Autodesk Fusion 360 part; units mm, degrees
(part 4 of 8)
  spline S98 degree 5 poles (306.7756, -389.774) (306.6868, -389.747) (306.5093, -389.6931) (306.243, -389.6127) (305.8878, -389.5066) (305.4436, -389.3756) (304.9994, -389.2464) (304.5549, -389.1189) (304.1104, -388.9931) (303.6657, -388.869) (303.2209, -388.7467) (302.776, -388.6262) (302.3309, -388.5074) (301.8858, -388.3905) (301.4405, -388.2753) (300.9951, -388.162) (300.5496, -388.0505) (300.1041, -387.9408) (299.6584, -387.833) (299.2127, -387.7271) (298.7668, -387.623) (298.3209, -387.5209) (297.875, -387.4207) (297.4289, -387.3224) (296.9828, -387.2261) (296.5366, -387.1317) (296.0904, -387.0393) (295.6441, -386.949) (295.1978, -386.8606) (294.7515, -386.7743) (294.3051, -386.6901) (293.8587, -386.6079) (293.4123, -386.5279) (292.9659, -386.45) (292.5194, -386.3742) (292.073, -386.3006) (291.6266, -386.2292) (291.1802, -386.1601) (290.7338, -386.0932) (290.2874, -386.0286) (289.8411, -385.9663) (289.3949, -385.9064) (288.9486, -385.8488) (288.5025, -385.7937) (288.0564, -385.741) (287.6104, -385.6908) (287.1645, -385.6431) (286.7186, -385.5981) (286.273, -385.5557) (285.8274, -385.5159) (285.3819, -385.4789) (284.9366, -385.4446) (284.4915, -385.4131) (284.0465, -385.3845) (283.6017, -385.3588) (283.1571, -385.3362) (282.7128, -385.3169) (282.2687, -385.3009) (281.825, -385.2883) (281.3815, -385.2792) (280.9383, -385.2735) (280.4954, -385.2712) (280.0528, -385.2725) (279.6543, -385.277) (279.3446, -385.2831) (279.1234, -385.2889) (278.9906, -385.2929) (278.9461, -385.2943) knots -1 -1 -1 -1 -1 -1 -0.98571429 -0.97142857 -0.95714286 -0.94285714 -0.92857143 -0.91428571 -0.9 -0.88571429 -0.87142857 -0.85714286 -0.84285714 -0.82857143 -0.81428571 -0.8 -0.78571429 -0.77142857 -0.75714286 -0.74285714 -0.72857143 -0.71428571 -0.7 -0.68571429 -0.67142857 -0.65714286 -0.64285714 -0.62857143 -0.61428571 -0.6 -0.58571429 -0.57142857 -0.55714286 -0.54285714 -0.52857143 -0.51428571 -0.5 -0.48571429 -0.47142857 -0.45714286 -0.44285714 -0.42857143 -0.41428571 -0.4 -0.38571429 -0.37142857 -0.35714286 -0.34285714 -0.32857143 -0.31428571 -0.3 -0.28571429 -0.27142857 -0.25714286 -0.24285714 -0.22857143 -0.21428571 -0.2 -0.18571429 -0.17142857 -0.15714286 -0.14285714 -0.12857143 -0.11428571 -0.10707295 -0.10707295 -0.10707295 -0.10707295 -0.10707295 -0.10707295
  spline S99 degree 3 poles (277.3377, -384.0136) (277.3775, -384.2165) (277.4566, -384.4096) (277.6843, -384.7546) (277.8308, -384.9033) (278.1397, -385.1137) (278.2917, -385.1853) (278.6124, -385.2786) (278.7791, -385.2997) (278.9461, -385.2943) knots 0 0 0 0 0.062015 0.062015 0.12403 0.12403 0.174133 0.174133 0.224236 0.224236 0.224236 0.224236
  arc A50 (277.3377, -384.0136) -> (275.5948, -375.8142) centre (11.949, -436.1388) ccw
  spline S100 degree 3 poles (276.5432, -373.99) (276.3518, -374.068) (276.1774, -374.1826) (275.8825, -374.4723) (275.7647, -374.6446) (275.6175, -374.9881) (275.5763, -375.151) (275.5463, -375.4837) (275.5576, -375.6514) (275.5948, -375.8142) knots 0 0 0 0 0.062015 0.062015 0.12403 0.12403 0.174133 0.174133 0.224236 0.224236 0.224236 0.224236
  spline S101 degree 5 poles (276.5432, -373.99) (276.5845, -373.9731) (276.7075, -373.9228) (276.9119, -373.8381) (277.1973, -373.7177) (277.5632, -373.5598) (277.968, -373.3809) (278.3717, -373.1987) (278.7743, -373.0133) (279.1757, -372.8245) (279.576, -372.6325) (279.9752, -372.4373) (280.3732, -372.2389) (280.7702, -372.0374) (281.1661, -371.8331) (281.5609, -371.6259) (281.9548, -371.4161) (282.3476, -371.2036) (282.7395, -370.9886) (283.1304, -370.7711) (283.5203, -370.5511) (283.9093, -370.3286) (284.2972, -370.1037) (284.6843, -369.8764) (285.0703, -369.6468) (285.4555, -369.415) (285.8397, -369.1809) (286.223, -368.9446) (286.6054, -368.7062) (286.9869, -368.4656) (287.3675, -368.223) (287.7472, -367.9783) (288.126, -367.7315) (288.5039, -367.4827) (288.8809, -367.2319) (289.2571, -366.9791) (289.6324, -366.7244) (290.0067, -366.4678) (290.3803, -366.2093) (290.7529, -365.9489) (291.1247, -365.6867) (291.4956, -365.4226) (291.8657, -365.1567) (292.2349, -364.889) (292.6033, -364.6196) (292.9708, -364.3484) (293.3374, -364.0754) (293.7033, -363.8008) (294.0682, -363.5244) (294.4324, -363.2463) (294.7956, -362.9666) (295.1581, -362.6851) (295.5197, -362.4021) (295.8805, -362.1174) (296.2404, -361.8311) (296.5995, -361.5432) (296.9578, -361.2537) (297.3152, -360.9626) (297.6718, -360.67) (298.0276, -360.3758) (298.3825, -360.08) (298.7367, -359.7828) (299.09, -359.484) (299.4424, -359.1837) (299.7238, -358.9423) (299.9344, -358.7605) (300.0746, -358.6391) (300.1447, -358.5783) knots 0.10707295 0.10707295 0.10707295 0.10707295 0.10707295 0.10707295 0.11428571 0.12857143 0.14285714 0.15714286 0.17142857 0.18571429 0.2 0.21428571 0.22857143 0.24285714 0.25714286 0.27142857 0.28571429 0.3 0.31428571 0.32857143 0.34285714 0.35714286 0.37142857 0.38571429 0.4 0.41428571 0.42857143 0.44285714 0.45714286 0.47142857 0.48571429 0.5 0.51428571 0.52857143 0.54285714 0.55714286 0.57142857 0.58571429 0.6 0.61428571 0.62857143 0.64285714 0.65714286 0.67142857 0.68571429 0.7 0.71428571 0.72857143 0.74285714 0.75714286 0.77142857 0.78571429 0.8 0.81428571 0.82857143 0.84285714 0.85714286 0.87142857 0.88571429 0.9 0.91428571 0.92857143 0.94285714 0.95714286 0.97142857 0.98571429 1 1 1 1 1 1
  arc A51 (300.1447, -358.5783) -> (297.4536, -349.1933) centre (11.949, -436.1388) ccw
  spline S102 degree 5 poles (297.4536, -349.1933) (297.362, -349.1789) (297.1787, -349.1502) (296.9037, -349.1077) (296.5372, -349.052) (296.0792, -348.9842) (295.6212, -348.918) (295.1634, -348.8536) (294.7057, -348.7909) (294.2481, -348.7299) (293.7906, -348.6707) (293.3332, -348.6133) (292.8759, -348.5576) (292.4188, -348.5037) (291.9619, -348.4517) (291.5051, -348.4014) (291.0484, -348.353) (290.5919, -348.3064) (290.1356, -348.2617) (289.6794, -348.2188) (289.2235, -348.1779) (288.7677, -348.1388) (288.3121, -348.1016) (287.8567, -348.0664) (287.4015, -348.033) (286.9466, -348.0017) (286.4918, -347.9723) (286.0373, -347.9449) (285.5831, -347.9196) (285.1291, -347.8962) (284.6753, -347.8749) (284.2218, -347.8557) (283.7686, -347.8386) (283.3157, -347.8235) (282.8631, -347.8107) (282.4107, -347.7999) (281.9587, -347.7914) (281.507, -347.785) (281.0557, -347.7809) (280.6047, -347.7791) (280.154, -347.7795) (279.7038, -347.7823) (279.2539, -347.7874) (278.8044, -347.7948) (278.3553, -347.8047) (277.9067, -347.8171) (277.4584, -347.832) (277.0107, -347.8494) (276.5634, -347.8694) (276.1167, -347.8921) (275.6704, -347.9174) (275.2247, -347.9455) (274.7795, -347.9762) (274.3349, -348.0098) (273.8908, -348.0463) (273.4474, -348.0858) (273.0047, -348.1284) (272.5627, -348.1744) (272.1215, -348.2237) (271.6811, -348.2764) (271.2414, -348.3324) (270.8025, -348.3918) (270.3644, -348.4547) (269.9705, -348.5146) (269.6646, -348.5637) (269.4464, -348.6003) (269.3154, -348.6227) (269.2715, -348.6304) knots -1 -1 -1 -1 -1 -1 -0.98571429 -0.97142857 -0.95714286 -0.94285714 -0.92857143 -0.91428571 -0.9 -0.88571429 -0.87142857 -0.85714286 -0.84285714 -0.82857143 -0.81428571 -0.8 -0.78571429 -0.77142857 -0.75714286 -0.74285714 -0.72857143 -0.71428571 -0.7 -0.68571429 -0.67142857 -0.65714286 -0.64285714 -0.62857143 -0.61428571 -0.6 -0.58571429 -0.57142857 -0.55714286 -0.54285714 -0.52857143 -0.51428571 -0.5 -0.48571429 -0.47142857 -0.45714286 -0.44285714 -0.42857143 -0.41428571 -0.4 -0.38571429 -0.37142857 -0.35714286 -0.34285714 -0.32857143 -0.31428571 -0.3 -0.28571429 -0.27142857 -0.25714286 -0.24285714 -0.22857143 -0.21428571 -0.2 -0.18571429 -0.17142857 -0.15714286 -0.14285714 -0.12857143 -0.11428571 -0.10707295 -0.10707295 -0.10707295 -0.10707295 -0.10707295 -0.10707295
  spline S103 degree 3 poles (267.5005, -347.5859) (267.5682, -347.7812) (267.6734, -347.9615) (267.9469, -348.2715) (268.1127, -348.3983) (268.4478, -348.5637) (268.6083, -348.6135) (268.9389, -348.6612) (269.1069, -348.6589) (269.2715, -348.6304) knots 0 0 0 0 0.062015 0.062015 0.12403 0.12403 0.174133 0.174133 0.224236 0.224236 0.224236 0.224236
  arc A52 (267.5005, -347.5859) -> (264.6335, -339.7088) centre (11.949, -436.1388) ccw
  spline S104 degree 3 poles (265.3188, -337.7704) (265.1401, -337.8743) (264.9834, -338.0121) (264.7316, -338.34) (264.6389, -338.527) (264.5409, -338.8877) (264.5228, -339.0547) (264.5394, -339.3883) (264.5739, -339.5528) (264.6335, -339.7088) knots 0 0 0 0 0.062015 0.062015 0.12403 0.12403 0.174133 0.174133 0.224236 0.224236 0.224236 0.224236
  spline S105 degree 5 poles (265.3188, -337.7704) (265.3573, -337.748) (265.4721, -337.681) (265.6628, -337.5687) (265.9286, -337.4098) (266.2689, -337.2025) (266.6449, -336.969) (267.0193, -336.7324) (267.3922, -336.4927) (267.7634, -336.2499) (268.1331, -336.0041) (268.5012, -335.7552) (268.8678, -335.5033) (269.2328, -335.2486) (269.5964, -334.9911) (269.9586, -334.731) (270.3194, -334.4684) (270.6789, -334.2034) (271.037, -333.9359) (271.3939, -333.6661) (271.7494, -333.394) (272.1036, -333.1195) (272.4565, -332.8428) (272.8081, -332.5639) (273.1585, -332.2828) (273.5076, -331.9996) (273.8555, -331.7143) (274.2022, -331.427) (274.5477, -331.1377) (274.892, -330.8464) (275.2351, -330.5531) (275.5771, -330.2579) (275.9178, -329.9608) (276.2574, -329.6618) (276.5959, -329.361) (276.9332, -329.0583) (277.2693, -328.7539) (277.6044, -328.4477) (277.9383, -328.1397) (278.2711, -327.83) (278.6028, -327.5186) (278.9333, -327.2054) (279.2628, -326.8906) (279.5912, -326.5742) (279.9184, -326.2561) (280.2446, -325.9364) (280.5697, -325.615) (280.8937, -325.2921) (281.2167, -324.9676) (281.5386, -324.6416) (281.8594, -324.314) (282.1791, -323.9849) (282.4978, -323.6543) (282.8155, -323.3222) (283.1321, -322.9885) (283.4476, -322.6535) (283.7621, -322.3169) (284.0755, -321.9789) (284.388, -321.6395) (284.6993, -321.2986) (285.0097, -320.9564) (285.319, -320.6127) (285.6273, -320.2677) (285.9345, -319.9213) (286.1795, -319.6431) (286.3628, -319.4338) (286.4848, -319.294) (286.5457, -319.224) knots 0.10707295 0.10707295 0.10707295 0.10707295 0.10707295 0.10707295 0.11428571 0.12857143 0.14285714 0.15714286 0.17142857 0.18571429 0.2 0.21428571 0.22857143 0.24285714 0.25714286 0.27142857 0.28571429 0.3 0.31428571 0.32857143 0.34285714 0.35714286 0.37142857 0.38571429 0.4 0.41428571 0.42857143 0.44285714 0.45714286 0.47142857 0.48571429 0.5 0.51428571 0.52857143 0.54285714 0.55714286 0.57142857 0.58571429 0.6 0.61428571 0.62857143 0.64285714 0.65714286 0.67142857 0.68571429 0.7 0.71428571 0.72857143 0.74285714 0.75714286 0.77142857 0.78571429 0.8 0.81428571 0.82857143 0.84285714 0.85714286 0.87142857 0.88571429 0.9 0.91428571 0.92857143 0.94285714 0.95714286 0.97142857 0.98571429 1 1 1 1 1 1
  arc A53 (286.5457, -319.224) -> (282.5747, -310.3049) centre (11.949, -436.1388) ccw
  spline S106 degree 5 poles (282.5747, -310.3049) (282.4819, -310.3034) (282.2964, -310.3005) (282.0182, -310.2966) (281.6475, -310.2925) (281.1845, -310.2891) (280.7218, -310.2873) (280.2594, -310.2872) (279.7974, -310.2888) (279.3358, -310.2921) (278.8745, -310.2972) (278.4136, -310.304) (277.953, -310.3125) (277.4929, -310.3227) (277.0331, -310.3348) (276.5738, -310.3486) (276.1148, -310.3642) (275.6563, -310.3816) (275.1982, -310.4008) (274.7405, -310.4219) (274.2833, -310.4447) (273.8265, -310.4695) (273.3701, -310.4961) (272.9143, -310.5245) (272.4589, -310.5549) (272.004, -310.5872) (271.5496, -310.6214) (271.0957, -310.6575) (270.6424, -310.6956) (270.1895, -310.7357) (269.7372, -310.7777) (269.2855, -310.8218) (268.8343, -310.8679) (268.3837, -310.9161) (267.9337, -310.9663) (267.4842, -311.0186) (267.0354, -311.0731) (266.5873, -311.1296) (266.1397, -311.1884) (265.6929, -311.2493) (265.2467, -311.3125) (264.8012, -311.3779) (264.3564, -311.4456) (263.9123, -311.5155) (263.4689, -311.5878) (263.0264, -311.6625) (262.5846, -311.7396) (262.1436, -311.8192) (261.7035, -311.9013) (261.2643, -311.9859) (260.8259, -312.0731) (260.3884, -312.1629) (259.9518, -312.2553) (259.5162, -312.3504) (259.0815, -312.4483) (258.6479, -312.5491) (258.2155, -312.653) (257.7842, -312.76) (257.3541, -312.8703) (256.9253, -312.9837) (256.4977, -313.1004) (256.0713, -313.2203) (255.6462, -313.3435) (255.2645, -313.4577) (254.9684, -313.5489) (254.7574, -313.6155) (254.6309, -313.656) (254.5884, -313.6696) knots -1 -1 -1 -1 -1 -1 -0.98571429 -0.97142857 -0.95714286 -0.94285714 -0.92857143 -0.91428571 -0.9 -0.88571429 -0.87142857 -0.85714286 -0.84285714 -0.82857143 -0.81428571 -0.8 -0.78571429 -0.77142857 -0.75714286 -0.74285714 -0.72857143 -0.71428571 -0.7 -0.68571429 -0.67142857 -0.65714286 -0.64285714 -0.62857143 -0.61428571 -0.6 -0.58571429 -0.57142857 -0.55714286 -0.54285714 -0.52857143 -0.51428571 -0.5 -0.48571429 -0.47142857 -0.45714286 -0.44285714 -0.42857143 -0.41428571 -0.4 -0.38571429 -0.37142857 -0.35714286 -0.34285714 -0.32857143 -0.31428571 -0.3 -0.28571429 -0.27142857 -0.25714286 -0.24285714 -0.22857143 -0.21428571 -0.2 -0.18571429 -0.17142857 -0.15714286 -0.14285714 -0.12857143 -0.11428571 -0.10707295 -0.10707295 -0.10707295 -0.10707295 -0.10707295 -0.10707295
  spline S107 degree 3 poles (252.6893, -312.8818) (252.7835, -313.0658) (252.9128, -313.2297) (253.2268, -313.4986) (253.4086, -313.6011) (253.7635, -313.7182) (253.9293, -313.7452) (254.2634, -313.7465) (254.4294, -313.7207) (254.5884, -313.6696) knots 0 0 0 0 0.062015 0.062015 0.12403 0.12403 0.174133 0.174133 0.224236 0.224236 0.224236 0.224236
  arc A54 (252.6893, -312.8818) -> (248.7539, -305.4804) centre (11.949, -436.1388) ccw
  spline S108 degree 3 poles (249.1628, -303.4654) (249.0003, -303.5932) (248.8643, -303.7515) (248.6606, -304.1113) (248.5948, -304.3093) (248.548, -304.6801) (248.5533, -304.8481) (248.6161, -305.1761) (248.6732, -305.3342) (248.7539, -305.4804) knots 0 0 0 0 0.062015 0.062015 0.12403 0.12403 0.174133 0.174133 0.224236 0.224236 0.224236 0.224236
  spline S109 degree 5 poles (249.1628, -303.4654) (249.1978, -303.4379) (249.3022, -303.3556) (249.4753, -303.2179) (249.7165, -303.0235) (250.0246, -302.7708) (250.3645, -302.4873) (250.7023, -302.2009) (251.0382, -301.9116) (251.372, -301.6196) (251.7039, -301.3247) (252.0338, -301.027) (252.3617, -300.7265) (252.6878, -300.4235) (253.012, -300.1179) (253.3345, -299.8099) (253.6552, -299.4996) (253.9743, -299.1871) (254.2917, -298.8725) (254.6075, -298.5556) (254.9217, -298.2366) (255.2342, -297.9156) (255.5452, -297.5924) (255.8546, -297.2673) (256.1624, -296.9402) (256.4688, -296.6111) (256.7736, -296.2802) (257.0769, -295.9474) (257.3788, -295.6129) (257.6792, -295.2765) (257.9782, -294.9383) (258.2757, -294.5984) (258.5718, -294.2568) (258.8665, -293.9134) (259.1598, -293.5684) (259.4517, -293.2218) (259.7422, -292.8735) (260.0313, -292.5236) (260.3191, -292.1722) (260.6056, -291.8192) (260.8907, -291.4646) (261.1745, -291.1085) (261.4569, -290.7509) (261.738, -290.3919) (262.0179, -290.0313) (262.2964, -289.6693) (262.5736, -289.3059) (262.8495, -288.941) (263.1242, -288.5747) (263.3975, -288.2071) (263.6696, -287.838) (263.9405, -287.4676) (264.2101, -287.0959) (264.4784, -286.7228) (264.7455, -286.3483) (265.0113, -285.9726) (265.2759, -285.5955) (265.5392, -285.2172) (265.8014, -284.8376) (266.0623, -284.4567) (266.322, -284.0746) (266.5804, -283.6913) (266.8377, -283.3067) (267.0938, -282.9209) (267.2976, -282.6113) (267.45, -282.3785) (267.5513, -282.2231) (267.6019, -282.1453) knots 0.10707295 0.10707295 0.10707295 0.10707295 0.10707295 0.10707295 0.11428571 0.12857143 0.14285714 0.15714286 0.17142857 0.18571429 0.2 0.21428571 0.22857143 0.24285714 0.25714286 0.27142857 0.28571429 0.3 0.31428571 0.32857143 0.34285714 0.35714286 0.37142857 0.38571429 0.4 0.41428571 0.42857143 0.44285714 0.45714286 0.47142857 0.48571429 0.5 0.51428571 0.52857143 0.54285714 0.55714286 0.57142857 0.58571429 0.6 0.61428571 0.62857143 0.64285714 0.65714286 0.67142857 0.68571429 0.7 0.71428571 0.72857143 0.74285714 0.75714286 0.77142857 0.78571429 0.8 0.81428571 0.82857143 0.84285714 0.85714286 0.87142857 0.88571429 0.9 0.91428571 0.92857143 0.94285714 0.95714286 0.97142857 0.98571429 1 1 1 1 1 1
  arc A55 (267.6019, -282.1453) -> (262.4283, -273.8657) centre (11.949, -436.1388) ccw
  spline S110 degree 5 poles (262.4283, -273.8657) (262.3362, -273.8771) (262.1521, -273.9) (261.8761, -273.935) (261.5084, -273.9825) (261.0494, -274.0435) (260.591, -274.1061) (260.1331, -274.1704) (259.6758, -274.2363) (259.2191, -274.3038) (258.763, -274.373) (258.3076, -274.4439) (257.8527, -274.5164) (257.3984, -274.5906) (256.9448, -274.6665) (256.4919, -274.7441) (256.0395, -274.8235) (255.5879, -274.9045) (255.1369, -274.9873) (254.6866, -275.0718) (254.237, -275.1581) (253.7881, -275.2462) (253.3399, -275.336) (252.8925, -275.4277) (252.4457, -275.5211) (251.9998, -275.6164) (251.5546, -275.7135) (251.1101, -275.8124) (250.6665, -275.9133) (250.2236, -276.016) (249.7816, -276.1206) (249.3403, -276.2271) (248.9, -276.3355) (248.4604, -276.4459) (248.0218, -276.5583) (247.584, -276.6727) (247.1472, -276.789) (246.7112, -276.9074) (246.2762, -277.0279) (245.8422, -277.1504) (245.4091, -277.2751) (244.9771, -277.4018) (244.546, -277.5307) (244.116, -277.6618) (243.687, -277.7951) (243.2592, -277.9307) (242.8324, -278.0685) (242.4068, -278.2087) (241.9824, -278.3512) (241.5592, -278.4961) (241.1372, -278.6435) (240.7165, -278.7933) (240.297, -278.9456) (239.8788, -279.1004) (239.4621, -279.2579) (239.0467, -279.418) (238.6329, -279.5811) (238.2207, -279.7471) (237.8102, -279.9161) (237.4014, -280.0881) (236.9941, -280.2632) (236.5886, -280.4413) (236.1848, -280.6225) (235.8227, -280.7887) (235.5422, -280.9202) (235.3425, -281.0155) (235.2228, -281.0732) (235.1827, -281.0926) knots -1 -1 -1 -1 -1 -1 -0.98571429 -0.97142857 -0.95714286 -0.94285714 -0.92857143 -0.91428571 -0.9 -0.88571429 -0.87142857 -0.85714286 -0.84285714 -0.82857143 -0.81428571 -0.8 -0.78571429 -0.77142857 -0.75714286 -0.74285714 -0.72857143 -0.71428571 -0.7 -0.68571429 -0.67142857 -0.65714286 -0.64285714 -0.62857143 -0.61428571 -0.6 -0.58571429 -0.57142857 -0.55714286 -0.54285714 -0.52857143 -0.51428571 -0.5 -0.48571429 -0.47142857 -0.45714286 -0.44285714 -0.42857143 -0.41428571 -0.4 -0.38571429 -0.37142857 -0.35714286 -0.34285714 -0.32857143 -0.31428571 -0.3 -0.28571429 -0.27142857 -0.25714286 -0.24285714 -0.22857143 -0.21428571 -0.2 -0.18571429 -0.17142857 -0.15714286 -0.14285714 -0.12857143 -0.11428571 -0.10707295 -0.10707295 -0.10707295 -0.10707295 -0.10707295 -0.10707295
  spline S111 degree 3 poles (233.1924, -280.5768) (233.3113, -280.7459) (233.4621, -280.8901) (233.8105, -281.1127) (234.0048, -281.1889) (234.3725, -281.2555) (234.5405, -281.2592) (234.8715, -281.2139) (235.0323, -281.1654) (235.1827, -281.0926) knots 0 0 0 0 0.062015 0.062015 0.12403 0.12403 0.174133 0.174133 0.224236 0.224236 0.224236 0.224236
  arc A56 (233.1924, -280.5768) -> (228.2652, -273.7951) centre (11.949, -436.1388) ccw
  spline S112 degree 3 poles (228.3897, -271.7428) (228.2465, -271.892) (228.1339, -272.0676) (227.9822, -272.4523) (227.9447, -272.6575) (227.9499, -273.0312) (227.9786, -273.1968) (228.0864, -273.5129) (228.165, -273.6615) (228.2652, -273.7951) knots 0 0 0 0 0.062015 0.062015 0.12403 0.12403 0.174133 0.174133 0.224236 0.224236 0.224236 0.224236
  spline S113 degree 5 poles (228.3897, -271.7428) (228.4205, -271.7107) (228.5124, -271.6147) (228.6647, -271.4542) (228.8765, -271.2281) (229.1465, -270.935) (229.4436, -270.607) (229.7382, -270.2763) (230.0306, -269.9431) (230.3205, -269.6074) (230.6081, -269.2692) (230.8934, -268.9285) (231.1763, -268.5854) (231.457, -268.2399) (231.7355, -267.8921) (232.012, -267.5423) (232.2865, -267.1904) (232.5589, -266.8365) (232.8295, -266.4807) (233.0981, -266.123) (233.3648, -265.7634) (233.6297, -265.402) (233.8926, -265.0387) (234.1537, -264.6737) (234.4131, -264.3069) (234.6706, -263.9384) (234.9264, -263.5683) (235.1805, -263.1966) (235.4329, -262.8232) (235.6835, -262.4483) (235.9325, -262.0718) (236.1798, -261.6938) (236.4255, -261.3143) (236.6695, -260.9333) (236.912, -260.5508) (237.1528, -260.1669) (237.392, -259.7816) (237.6297, -259.3949) (237.8657, -259.0068) (238.1003, -258.6174) (238.3333, -258.2266) (238.5647, -257.8345) (238.7946, -257.4411) (239.0231, -257.0464) (239.25, -256.6504) (239.4754, -256.2531) (239.6993, -255.8546) (239.9218, -255.4549) (240.1428, -255.054) (240.3624, -254.6519) (240.5804, -254.2485) (240.7971, -253.844) (241.0123, -253.4384) (241.2261, -253.0316) (241.4385, -252.6236) (241.6494, -252.2145) (241.859, -251.8043) (242.0671, -251.393) (242.2739, -250.9806) (242.4792, -250.5672) (242.6832, -250.1526) (242.8858, -249.737) (243.087, -249.3204) (243.2869, -248.9027) (243.4457, -248.5677) (243.5642, -248.316) (243.6429, -248.148) (243.6822, -248.064) knots 0.10707295 0.10707295 0.10707295 0.10707295 0.10707295 0.10707295 0.11428571 0.12857143 0.14285714 0.15714286 0.17142857 0.18571429 0.2 0.21428571 0.22857143 0.24285714 0.25714286 0.27142857 0.28571429 0.3 0.31428571 0.32857143 0.34285714 0.35714286 0.37142857 0.38571429 0.4 0.41428571 0.42857143 0.44285714 0.45714286 0.47142857 0.48571429 0.5 0.51428571 0.52857143 0.54285714 0.55714286 0.57142857 0.58571429 0.6 0.61428571 0.62857143 0.64285714 0.65714286 0.67142857 0.68571429 0.7 0.71428571 0.72857143 0.74285714 0.75714286 0.77142857 0.78571429 0.8 0.81428571 0.82857143 0.84285714 0.85714286 0.87142857 0.88571429 0.9 0.91428571 0.92857143 0.94285714 0.95714286 0.97142857 0.98571429 1 1 1 1 1 1
  arc A57 (243.6822, -248.064) -> (237.4066, -240.585) centre (11.949, -436.1388) ccw
  spline S114 degree 5 poles (237.4066, -240.585) (237.317, -240.6091) (237.1378, -240.6574) (236.8694, -240.7304) (236.5119, -240.8286) (236.0659, -240.9529) (235.6206, -241.0787) (235.1762, -241.2061) (234.7325, -241.335) (234.2897, -241.4654) (233.8476, -241.5974) (233.4064, -241.731) (232.9661, -241.8661) (232.5266, -242.0028) (232.0879, -242.1411) (231.6502, -242.281) (231.2133, -242.4225) (230.7773, -242.5657) (230.3423, -242.7104) (229.9081, -242.8568) (229.4749, -243.0048) (229.0426, -243.1545) (228.6113, -243.3058) (228.181, -243.4588) (227.7516, -243.6135) (227.3232, -243.77) (226.8958, -243.9281) (226.4695, -244.0879) (226.0442, -244.2495) (225.6199, -244.4129) (225.1968, -244.578) (224.7747, -244.7448) (224.3537, -244.9135) (223.9338, -245.084) (223.515, -245.2563) (223.0974, -245.4305) (222.681, -245.6066) (222.2658, -245.7845) (221.8518, -245.9643) (221.4391, -246.1461) (221.0276, -246.3298) (220.6173, -246.5154) (220.2084, -246.7031) (219.8008, -246.8927) (219.3946, -247.0844) (218.9897, -247.2782) (218.5863, -247.4741) (218.1844, -247.6721) (217.784, -247.8723) (217.385, -248.0748) (216.9877, -248.2794) (216.5919, -248.4863) (216.1977, -248.6955) (215.8051, -248.907) (215.4143, -249.1209) (215.0253, -249.3374) (214.6382, -249.5564) (214.2532, -249.7781) (213.8702, -250.0026) (213.4892, -250.2299) (213.1103, -250.4599) (212.7335, -250.6927) (212.3589, -250.9283) (212.0234, -251.1433) (211.7639, -251.3126) (211.5794, -251.4347) (211.4689, -251.5086) (211.4319, -251.5334) knots -1 -1 -1 -1 -1 -1 -0.98571429 -0.97142857 -0.95714286 -0.94285714 -0.92857143 -0.91428571 -0.9 -0.88571429 -0.87142857 -0.85714286 -0.84285714 -0.82857143 -0.81428571 -0.8 -0.78571429 -0.77142857 -0.75714286 -0.74285714 -0.72857143 -0.71428571 -0.7 -0.68571429 -0.67142857 -0.65714286 -0.64285714 -0.62857143 -0.61428571 -0.6 -0.58571429 -0.57142857 -0.55714286 -0.54285714 -0.52857143 -0.51428571 -0.5 -0.48571429 -0.47142857 -0.45714286 -0.44285714 -0.42857143 -0.41428571 -0.4 -0.38571429 -0.37142857 -0.35714286 -0.34285714 -0.32857143 -0.31428571 -0.3 -0.28571429 -0.27142857 -0.25714286 -0.24285714 -0.22857143 -0.21428571 -0.2 -0.18571429 -0.17142857 -0.15714286 -0.14285714 -0.12857143 -0.11428571 -0.10707295 -0.10707295 -0.10707295 -0.10707295 -0.10707295 -0.10707295
  spline S115 degree 3 poles (209.3892, -251.2996) (209.5305, -251.4505) (209.6999, -251.5723) (210.0759, -251.7443) (210.2789, -251.7927) (210.6523, -251.8075) (210.8192, -251.7877) (211.1406, -251.6969) (211.2932, -251.6263) (211.4319, -251.5334) knots 0 0 0 0 0.062015 0.062015 0.12403 0.12403 0.174133 0.174133 0.224236 0.224236 0.224236 0.224236
  arc A58 (209.3892, -251.2996) -> (203.5662, -245.2696) centre (11.949, -436.1388) ccw
  spline S116 degree 3 poles (203.4038, -243.22) (203.2828, -243.3876) (203.1957, -243.5772) (203.0991, -243.9792) (203.0905, -244.1877) (203.1476, -244.5571) (203.199, -244.7171) (203.3499, -245.0151) (203.4483, -245.1513) (203.5662, -245.2696) knots 0 0 0 0 0.062015 0.062015 0.12403 0.12403 0.174133 0.174133 0.224236 0.224236 0.224236 0.224236
  spline S117 degree 5 poles (203.4038, -243.22) (203.4299, -243.1839) (203.5075, -243.076) (203.636, -242.8959) (203.8142, -242.6425) (204.0408, -242.3147) (204.2894, -241.9485) (204.5351, -241.5801) (204.7783, -241.2095) (205.0187, -240.8367) (205.2564, -240.4617) (205.4915, -240.0846) (205.7239, -239.7054) (205.9538, -239.3242) (206.1812, -238.9411) (206.4063, -238.5562) (206.6291, -238.1695) (206.8497, -237.7812) (207.0681, -237.3912) (207.2843, -236.9996) (207.4984, -236.6064) (207.7103, -236.2116) (207.9202, -235.8153) (208.1279, -235.4175) (208.3337, -235.0182) (208.5375, -234.6174) (208.7393, -234.2153) (208.9391, -233.8118) (209.1371, -233.407) (209.3331, -233.0008) (209.5273, -232.5933) (209.7196, -232.1846) (209.9101, -231.7746) (210.0987, -231.3633) (210.2855, -230.9508) (210.4706, -230.5372) (210.6538, -230.1223) (210.8354, -229.7063) (211.0151, -229.2891) (211.1932, -228.8708) (211.3695, -228.4514) (211.5441, -228.0309) (211.7171, -227.6093) (211.8883, -227.1867) (212.0579, -226.763) (212.2259, -226.3382) (212.3922, -225.9124) (212.5569, -225.4856) (212.7199, -225.0579) (212.8814, -224.6291) (213.0412, -224.1993) (213.1994, -223.7686) (213.3561, -223.337) (213.5112, -222.9043) (213.6647, -222.4708) (213.8167, -222.0363) (213.9671, -221.601) (214.116, -221.1647) (214.2633, -220.7276) (214.4091, -220.2895) (214.5534, -219.8506) (214.6962, -219.4109) (214.8375, -218.9703) (214.9773, -218.5289) (215.0879, -218.1751) (215.1703, -217.9093) (215.2248, -217.732) (215.252, -217.6433) knots 0.10707295 0.10707295 0.10707295 0.10707295 0.10707295 0.10707295 0.11428571 0.12857143 0.14285714 0.15714286 0.17142857 0.18571429 0.2 0.21428571 0.22857143 0.24285714 0.25714286 0.27142857 0.28571429 0.3 0.31428571 0.32857143 0.34285714 0.35714286 0.37142857 0.38571429 0.4 0.41428571 0.42857143 0.44285714 0.45714286 0.47142857 0.48571429 0.5 0.51428571 0.52857143 0.54285714 0.55714286 0.57142857 0.58571429 0.6 0.61428571 0.62857143 0.64285714 0.65714286 0.67142857 0.68571429 0.7 0.71428571 0.72857143 0.74285714 0.75714286 0.77142857 0.78571429 0.8 0.81428571 0.82857143 0.84285714 0.85714286 0.87142857 0.88571429 0.9 0.91428571 0.92857143 0.94285714 0.95714286 0.97142857 0.98571429 1 1 1 1 1 1
  arc A59 (215.252, -217.6433) -> (207.9966, -211.1104) centre (11.949, -436.1388) ccw
  spline S118 degree 5 poles (207.9966, -211.1104) (207.9112, -211.1468) (207.7406, -211.2196) (207.4849, -211.3292) (207.1446, -211.4762) (206.7202, -211.6614) (206.2968, -211.848) (205.8743, -212.036) (205.4529, -212.2253) (205.0326, -212.4161) (204.6132, -212.6084) (204.1949, -212.802) (203.7776, -212.9971) (203.3614, -213.1937) (202.9463, -213.3917) (202.5323, -213.5911) (202.1194, -213.7921) (201.7076, -213.9945) (201.2969, -214.1984) (200.8873, -214.4037) (200.4789, -214.6106) (200.0717, -214.819) (199.6656, -215.0289) (199.2607, -215.2403) (198.8571, -215.4533) (198.4546, -215.6678) (198.0534, -215.8838) (197.6535, -216.1015) (197.2548, -216.3207) (196.8574, -216.5415) (196.4613, -216.7639) (196.0666, -216.9879) (195.6731, -217.2135) (195.2811, -217.4408) (194.8904, -217.6697) (194.5011, -217.9003) (194.1132, -218.1326) (193.7268, -218.3665) (193.3419, -218.6022) (192.9584, -218.8397) (192.5765, -219.0789) (192.1961, -219.3198) (191.8173, -219.5625) (191.4401, -219.8071) (191.0645, -220.0534) (190.6905, -220.3017) (190.3183, -220.5518) (189.9478, -220.8038) (189.5792, -221.0578) (189.2123, -221.3138) (188.8473, -221.5718) (188.4841, -221.8317) (188.1229, -222.0937) (187.7636, -222.3578) (187.4063, -222.6241) (187.0513, -222.8925) (186.6984, -223.1633) (186.348, -223.4365) (185.9999, -223.7121) (185.6543, -223.9902) (185.3112, -224.2707) (184.9704, -224.5537) (184.6322, -224.8391) (184.3299, -225.0987) (184.0965, -225.3025) (183.9308, -225.4491) (183.8317, -225.5376) (183.7985, -225.5673) knots -1 -1 -1 -1 -1 -1 -0.98571429 -0.97142857 -0.95714286 -0.94285714 -0.92857143 -0.91428571 -0.9 -0.88571429 -0.87142857 -0.85714286 -0.84285714 -0.82857143 -0.81428571 -0.8 -0.78571429 -0.77142857 -0.75714286 -0.74285714 -0.72857143 -0.71428571 -0.7 -0.68571429 -0.67142857 -0.65714286 -0.64285714 -0.62857143 -0.61428571 -0.6 -0.58571429 -0.57142857 -0.55714286 -0.54285714 -0.52857143 -0.51428571 -0.5 -0.48571429 -0.47142857 -0.45714286 -0.44285714 -0.42857143 -0.41428571 -0.4 -0.38571429 -0.37142857 -0.35714286 -0.34285714 -0.32857143 -0.31428571 -0.3 -0.28571429 -0.27142857 -0.25714286 -0.24285714 -0.22857143 -0.21428571 -0.2 -0.18571429 -0.17142857 -0.15714286 -0.14285714 -0.12857143 -0.11428571 -0.10707295 -0.10707295 -0.10707295 -0.10707295 -0.10707295 -0.10707295
  spline S119 degree 3 poles (181.7431, -225.62) (181.904, -225.7498) (182.0887, -225.8469) (182.485, -225.9649) (182.6927, -225.9846) (183.0646, -225.9472) (183.2271, -225.9044) (183.5328, -225.7697) (183.674, -225.6787) (183.7985, -225.5673) knots 0 0 0 0 0.062015 0.062015 0.12403 0.12403 0.174133 0.174133 0.224236 0.224236 0.224236 0.224236
  arc A60 (181.7431, -225.62) -> (175.1375, -220.4592) centre (11.949, -436.1388) ccw
  spline S120 degree 3 poles (174.6915, -218.4521) (174.595, -218.6349) (174.5351, -218.8348) (174.4954, -219.2464) (174.5159, -219.454) (174.6239, -219.8118) (174.6971, -219.9631) (174.8879, -220.2372) (175.0043, -220.3584) (175.1375, -220.4592) knots 0 0 0 0 0.062015 0.062015 0.12403 0.12403 0.174133 0.174133 0.224236 0.224236 0.224236 0.224236
  spline S121 degree 5 poles (174.6915, -218.4521) (174.7123, -218.4127) (174.7741, -218.2951) (174.8763, -218.0988) (175.0176, -217.8231) (175.1963, -217.467) (175.3914, -217.0698) (175.5836, -216.6707) (175.7727, -216.2698) (175.9589, -215.8672) (176.1422, -215.4629) (176.3225, -215.0567) (176.4998, -214.6489) (176.6744, -214.2394) (176.8463, -213.8283) (177.0157, -213.4158) (177.1825, -213.0019) (177.3469, -212.5867) (177.5089, -212.1701) (177.6685, -211.7522) (177.8258, -211.333) (177.9807, -210.9126) (178.1333, -210.4909) (178.2837, -210.068) (178.4319, -209.644) (178.5779, -209.2188) (178.7218, -208.7925) (178.8636, -208.3651) (179.0032, -207.9367) (179.1409, -207.5072) (179.2764, -207.0766) (179.41, -206.6451) (179.5415, -206.2126) (179.6711, -205.7791) (179.7987, -205.3446) (179.9244, -204.9092) (180.0481, -204.4729) (180.17, -204.0356) (180.2899, -203.5975) (180.408, -203.1585) (180.5243, -202.7186) (180.6387, -202.2779) (180.7513, -201.8364) (180.862, -201.394) (180.971, -200.9508) (181.0782, -200.5068) (181.1836, -200.062) (181.2873, -199.6165) (181.3892, -199.1702) (181.4894, -198.7231) (181.5879, -198.2753) (181.6847, -197.8267) (181.7797, -197.3775) (181.8731, -196.9275) (181.9648, -196.4768) (182.0548, -196.0254) (182.1432, -195.5734) (182.2299, -195.1206) (182.315, -194.6672) (182.3984, -194.2132) (182.4802, -193.7585) (182.5604, -193.3031) (182.639, -192.8472) (182.716, -192.3906) (182.7763, -192.0248) (182.8208, -191.7502) (182.8502, -191.567) (182.8648, -191.4753) knots 0.10707295 0.10707295 0.10707295 0.10707295 0.10707295 0.10707295 0.11428571 0.12857143 0.14285714 0.15714286 0.17142857 0.18571429 0.2 0.21428571 0.22857143 0.24285714 0.25714286 0.27142857 0.28571429 0.3 0.31428571 0.32857143 0.34285714 0.35714286 0.37142857 0.38571429 0.4 0.41428571 0.42857143 0.44285714 0.45714286 0.47142857 0.48571429 0.5 0.51428571 0.52857143 0.54285714 0.55714286 0.57142857 0.58571429 0.6 0.61428571 0.62857143 0.64285714 0.65714286 0.67142857 0.68571429 0.7 0.71428571 0.72857143 0.74285714 0.75714286 0.77142857 0.78571429 0.8 0.81428571 0.82857143 0.84285714 0.85714286 0.87142857 0.88571429 0.9 0.91428571 0.92857143 0.94285714 0.95714286 0.97142857 0.98571429 1 1 1 1 1 1
  arc A61 (182.8648, -191.4753) -> (174.7708, -186.0159) centre (11.949, -436.1388) ccw
  spline S122 degree 5 poles (174.7708, -186.0159) (174.6913, -186.0637) (174.5324, -186.1596) (174.2945, -186.3037) (173.978, -186.4967) (173.5835, -186.7391) (173.1901, -186.9828) (172.798, -187.2277) (172.407, -187.4739) (172.0173, -187.7214) (171.6288, -187.9701) (171.2415, -188.2201) (170.8555, -188.4714) (170.4707, -188.7239) (170.0871, -188.9778) (169.7049, -189.2329) (169.324, -189.4893) (168.9443, -189.7471) (168.566, -190.0061) (168.189, -190.2665) (167.8134, -190.5282) (167.4391, -190.7912) (167.0662, -191.0556) (166.6947, -191.3213) (166.3246, -191.5884) (165.956, -191.8568) (165.5887, -192.1266) (165.223, -192.3978) (164.8587, -192.6703) (164.4959, -192.9443) (164.1346, -193.2197) (163.7748, -193.4964) (163.4167, -193.7746) (163.06, -194.0542) (162.705, -194.3353) (162.3516, -194.6178) (161.9998, -194.9018) (161.6497, -195.1873) (161.3014, -195.4743) (160.9547, -195.7628) (160.6098, -196.0528) (160.2666, -196.3443) (159.9252, -196.6374) (159.5857, -196.9321) (159.2481, -197.2283) (158.9123, -197.5262) (158.5785, -197.8257) (158.2467, -198.1268) (157.917, -198.4296) (157.5893, -198.7342) (157.2638, -199.0404) (156.9403, -199.3484) (156.6191, -199.6582) (156.3, -199.9697) (155.9833, -200.283) (155.669, -200.5983) (155.3573, -200.9156) (155.0483, -201.2349) (154.742, -201.5562) (154.4385, -201.8797) (154.1377, -202.2052) (153.8396, -202.5329) (153.5444, -202.8626) (153.2812, -203.1618) (153.0785, -203.396) (152.9348, -203.5643) (152.8489, -203.6657) (152.8201, -203.6997) knots -1 -1 -1 -1 -1 -1 -0.98571429 -0.97142857 -0.95714286 -0.94285714 -0.92857143 -0.91428571 -0.9 -0.88571429 -0.87142857 -0.85714286 -0.84285714 -0.82857143 -0.81428571 -0.8 -0.78571429 -0.77142857 -0.75714286 -0.74285714 -0.72857143 -0.71428571 -0.7 -0.68571429 -0.67142857 -0.65714286 -0.64285714 -0.62857143 -0.61428571 -0.6 -0.58571429 -0.57142857 -0.55714286 -0.54285714 -0.52857143 -0.51428571 -0.5 -0.48571429 -0.47142857 -0.45714286 -0.44285714 -0.42857143 -0.41428571 -0.4 -0.38571429 -0.37142857 -0.35714286 -0.34285714 -0.32857143 -0.31428571 -0.3 -0.28571429 -0.27142857 -0.25714286 -0.24285714 -0.22857143 -0.21428571 -0.2 -0.18571429 -0.17142857 -0.15714286 -0.14285714 -0.12857143 -0.11428571 -0.10707295 -0.10707295 -0.10707295 -0.10707295 -0.10707295 -0.10707295
  spline S123 degree 3 poles (150.7922, -204.038) (150.9696, -204.1441) (151.166, -204.2146) (151.5748, -204.2762) (151.7833, -204.2668) (152.1463, -204.1781) (152.3013, -204.1131) (152.5852, -203.9372) (152.7124, -203.8273) (152.8201, -203.6997) knots 0 0 0 0 0.062015 0.062015 0.12403 0.12403 0.174133 0.174133 0.224236 0.224236 0.224236 0.224236
  arc A62 (150.7922, -204.038) -> (143.5326, -199.8467) centre (11.949, -436.1388) ccw
  spline S124 degree 3 poles (142.8115, -197.9213) (142.7414, -198.1157) (142.71, -198.322) (142.7279, -198.7351) (142.7771, -198.9379) (142.9338, -199.2771) (143.0274, -199.4168) (143.2545, -199.6617) (143.3867, -199.7654) (143.5326, -199.8467) knots 0 0 0 0 0.062015 0.062015 0.12403 0.12403 0.174133 0.174133 0.224236 0.224236 0.224236 0.224236
  spline S125 degree 5 poles (142.8115, -197.9213) (142.8267, -197.8793) (142.8716, -197.7543) (142.9454, -197.5457) (143.0469, -197.253) (143.1743, -196.8755) (143.3123, -196.4549) (143.447, -196.033) (143.5786, -195.6097) (143.7069, -195.1851) (143.8321, -194.7592) (143.9541, -194.3319) (144.073, -193.9033) (144.1889, -193.4735) (144.3019, -193.0426) (144.4122, -192.6105) (144.5198, -192.1774) (144.6248, -191.7433) (144.7272, -191.3083) (144.8271, -190.8722) (144.9245, -190.4352) (145.0195, -189.9973) (145.1119, -189.5585) (145.202, -189.1188) (145.2897, -188.6783) (145.3751, -188.2369) (145.4583, -187.7947) (145.5392, -187.3518) (145.6179, -186.9081) (145.6944, -186.4636) (145.7687, -186.0184) (145.8409, -185.5725) (145.911, -185.1258) (145.9789, -184.6785) (146.0448, -184.2305) (146.1087, -183.7819) (146.1705, -183.3326) (146.2303, -182.8826) (146.2882, -182.4321) (146.344, -181.9809) (146.3979, -181.5291) (146.4499, -181.0768) (146.4999, -180.6239) (146.548, -180.1704) (146.5943, -179.7163) (146.6386, -179.2617) (146.6811, -178.8066) (146.7218, -178.351) (146.7606, -177.8948) (146.7976, -177.4381) (146.8328, -176.981) (146.8662, -176.5233) (146.8978, -176.0652) (146.9276, -175.6066) (146.9557, -175.1476) (146.982, -174.688) (147.0066, -174.2281) (147.0295, -173.7677) (147.0506, -173.3068) (147.0701, -172.8456) (147.0878, -172.3839) (147.1039, -171.9219) (147.1182, -171.4594) (147.1309, -170.9965) (147.1398, -170.6259) (147.1456, -170.3478) (147.1492, -170.1623) (147.1509, -170.0695) knots 0.10707295 0.10707295 0.10707295 0.10707295 0.10707295 0.10707295 0.11428571 0.12857143 0.14285714 0.15714286 0.17142857 0.18571429 0.2 0.21428571 0.22857143 0.24285714 0.25714286 0.27142857 0.28571429 0.3 0.31428571 0.32857143 0.34285714 0.35714286 0.37142857 0.38571429 0.4 0.41428571 0.42857143 0.44285714 0.45714286 0.47142857 0.48571429 0.5 0.51428571 0.52857143 0.54285714 0.55714286 0.57142857 0.58571429 0.6 0.61428571 0.62857143 0.64285714 0.65714286 0.67142857 0.68571429 0.7 0.71428571 0.72857143 0.74285714 0.75714286 0.77142857 0.78571429 0.8 0.81428571 0.82857143 0.84285714 0.85714286 0.87142857 0.88571429 0.9 0.91428571 0.92857143 0.94285714 0.95714286 0.97142857 0.98571429 1 1 1 1 1 1
  arc A63 (147.1509, -170.0695) -> (138.3758, -165.7896) centre (11.949, -436.1388) ccw
  spline S126 degree 5 poles (138.3758, -165.7896) (138.3038, -165.8481) (138.1598, -165.9651) (137.9443, -166.141) (137.6576, -166.3761) (137.3007, -166.6711) (136.9451, -166.9671) (136.5909, -167.2642) (136.238, -167.5625) (135.8865, -167.8617) (135.5364, -168.1621) (135.1877, -168.4636) (134.8403, -168.7661) (134.4944, -169.0698) (134.15, -169.3745) (133.807, -169.6804) (133.4654, -169.9874) (133.1254, -170.2954) (132.7868, -170.6046) (132.4497, -170.9149) (132.1141, -171.2264) (131.7801, -171.5389) (131.4477, -171.8526) (131.1167, -172.1674) (130.7874, -172.4834) (130.4597, -172.8005) (130.1336, -173.1188) (129.8091, -173.4382) (129.4863, -173.7588) (129.1652, -174.0806) (128.8457, -174.4036) (128.528, -174.7277) (128.212, -175.0531) (127.8978, -175.3796) (127.5853, -175.7073) (127.2747, -176.0363) (126.9659, -176.3665) (126.6589, -176.6979) (126.3538, -177.0306) (126.0507, -177.3645) (125.7495, -177.6997) (125.4503, -178.0362) (125.153, -178.3739) (124.8578, -178.7129) (124.5646, -179.0533) (124.2736, -179.395) (123.9848, -179.738) (123.6981, -180.0824) (123.4137, -180.4282) (123.1316, -180.7754) (122.8519, -181.124) (122.5744, -181.474) (122.2994, -181.8254) (122.0268, -182.1783) (121.7568, -182.5327) (121.4895, -182.8886) (121.225, -183.2462) (120.9634, -183.6053) (120.7048, -183.9662) (120.4492, -184.3288) (120.1966, -184.693) (119.9471, -185.059) (119.7007, -185.4266) (119.4816, -185.7594) (119.3135, -186.0196) (119.1946, -186.2062) (119.1237, -186.3186) (119.0999, -186.3563) knots -1 -1 -1 -1 -1 -1 -0.98571429 -0.97142857 -0.95714286 -0.94285714 -0.92857143 -0.91428571 -0.9 -0.88571429 -0.87142857 -0.85714286 -0.84285714 -0.82857143 -0.81428571 -0.8 -0.78571429 -0.77142857 -0.75714286 -0.74285714 -0.72857143 -0.71428571 -0.7 -0.68571429 -0.67142857 -0.65714286 -0.64285714 -0.62857143 -0.61428571 -0.6 -0.58571429 -0.57142857 -0.55714286 -0.54285714 -0.52857143 -0.51428571 -0.5 -0.48571429 -0.47142857 -0.45714286 -0.44285714 -0.42857143 -0.41428571 -0.4 -0.38571429 -0.37142857 -0.35714286 -0.34285714 -0.32857143 -0.31428571 -0.3 -0.28571429 -0.27142857 -0.25714286 -0.24285714 -0.22857143 -0.21428571 -0.2 -0.18571429 -0.17142857 -0.15714286 -0.14285714 -0.12857143 -0.11428571 -0.10707295 -0.10707295 -0.10707295 -0.10707295 -0.10707295 -0.10707295
  spline S127 degree 3 poles (117.1388, -186.9736) (117.3292, -187.054) (117.5335, -187.0964) (117.9469, -187.1006) (118.1521, -187.0622) (118.4992, -186.9238) (118.6436, -186.8379) (118.9003, -186.6242) (119.011, -186.4977) (119.0999, -186.3563) knots 0 0 0 0 0.062015 0.062015 0.12403 0.12403 0.174133 0.174133 0.224236 0.224236 0.224236 0.224236
  arc A64 (117.1388, -186.9736) -> (109.3665, -183.8334) centre (11.949, -436.1388) ccw
  spline S128 degree 3 poles (108.3845, -182.027) (108.3422, -182.2294) (108.3397, -182.438) (108.4149, -182.8446) (108.4919, -183.0385) (108.6943, -183.3527) (108.8064, -183.4779) (109.0654, -183.6889) (109.2107, -183.7732) (109.3665, -183.8334) knots 0 0 0 0 0.062015 0.062015 0.12403 0.12403 0.174133 0.174133 0.224236 0.224236 0.224236 0.224236
  spline S129 degree 5 poles (108.3845, -182.027) (108.3937, -181.9834) (108.4207, -181.8533) (108.4648, -181.6365) (108.5246, -181.3325) (108.5983, -180.9409) (108.6764, -180.5053) (108.751, -180.0687) (108.8224, -179.6313) (108.8904, -179.1929) (108.9551, -178.7537) (109.0164, -178.3136) (109.0745, -177.8726) (109.1295, -177.4309) (109.1814, -176.9884) (109.2305, -176.5452) (109.2768, -176.1014) (109.3203, -175.6569) (109.3612, -175.2118) (109.3995, -174.7661) (109.4351, -174.3198) (109.4682, -173.8729) (109.4987, -173.4255) (109.5267, -172.9776) (109.5522, -172.5291) (109.5754, -172.0801) (109.5962, -171.6307) (109.6146, -171.1808) (109.6308, -170.7304) (109.6447, -170.2797) (109.6564, -169.8284) (109.6658, -169.3768) (109.673, -168.9248) (109.6781, -168.4723) (109.681, -168.0195) (109.6818, -167.5664) (109.6805, -167.1128) (109.6771, -166.6589) (109.6716, -166.2047) (109.6641, -165.7502) (109.6546, -165.2953) (109.6431, -164.8401) (109.6297, -164.3846) (109.6142, -163.9289) (109.5968, -163.4728) (109.5775, -163.0165) (109.5562, -162.5599) (109.5331, -162.103) (109.508, -161.6459) (109.4811, -161.1885) (109.4523, -160.7309) (109.4217, -160.2731) (109.3893, -159.815) (109.355, -159.3567) (109.3189, -158.8982) (109.281, -158.4395) (109.2413, -157.9806) (109.1999, -157.5215) (109.1567, -157.0622) (109.1118, -156.6027) (109.0651, -156.1431) (109.0167, -155.6833) (108.9665, -155.2233) (108.9147, -154.7632) (108.8718, -154.395) (108.8389, -154.1187) (108.8167, -153.9345) (108.8054, -153.8424) knots 0.10707295 0.10707295 0.10707295 0.10707295 0.10707295 0.10707295 0.11428571 0.12857143 0.14285714 0.15714286 0.17142857 0.18571429 0.2 0.21428571 0.22857143 0.24285714 0.25714286 0.27142857 0.28571429 0.3 0.31428571 0.32857143 0.34285714 0.35714286 0.37142857 0.38571429 0.4 0.41428571 0.42857143 0.44285714 0.45714286 0.47142857 0.48571429 0.5 0.51428571 0.52857143 0.54285714 0.55714286 0.57142857 0.58571429 0.6 0.61428571 0.62857143 0.64285714 0.65714286 0.67142857 0.68571429 0.7 0.71428571 0.72857143 0.74285714 0.75714286 0.77142857 0.78571429 0.8 0.81428571 0.82857143 0.84285714 0.85714286 0.87142857 0.88571429 0.9 0.91428571 0.92857143 0.94285714 0.95714286 0.97142857 0.98571429 1 1 1 1 1 1
  arc A65 (108.8054, -153.8424) -> (99.5201, -150.8254) centre (11.949, -436.1388) ccw
  spline S130 degree 5 poles (99.5201, -150.8254) (99.4569, -150.8933) (99.3306, -151.0293) (99.1416, -151.2334) (98.8905, -151.5061) (98.5781, -151.8479) (98.2672, -152.1906) (97.9578, -152.5341) (97.6499, -152.8785) (97.3434, -153.2238) (97.0385, -153.57) (96.7351, -153.9171) (96.4333, -154.265) (96.133, -154.6139) (95.8343, -154.9636) (95.5372, -155.3142) (95.2417, -155.6657) (94.9478, -156.0181) (94.6556, -156.3714) (94.365, -156.7256) (94.076, -157.0807) (93.7888, -157.4367) (93.5032, -157.7936) (93.2193, -158.1514) (92.9372, -158.5102) (92.6568, -158.8698) (92.3781, -159.2304) (92.1013, -159.5919) (91.8262, -159.9543) (91.553, -160.3176) (91.2816, -160.6819) (91.0121, -161.0471) (90.7444, -161.4132) (90.4787, -161.7803) (90.2149, -162.1484) (89.9531, -162.5174) (89.6932, -162.8873) (89.4354, -163.2582) (89.1796, -163.6301) (88.9259, -164.003) (88.6742, -164.3768) (88.4247, -164.7517) (88.1774, -165.1275) (87.9322, -165.5043) (87.6893, -165.8822) (87.4487, -166.261) (87.2103, -166.6409) (86.9744, -167.0219) (86.7409, -167.4039) (86.5099, -167.7869) (86.2814, -168.1711) (86.0553, -168.5563) (85.8319, -168.9425) (85.6111, -169.3299) (85.393, -169.7185) (85.1778, -170.1081) (84.9656, -170.499) (84.7566, -170.8911) (84.5507, -171.2845) (84.3481, -171.6791) (84.1487, -172.0749) (83.9525, -172.472) (83.7596, -172.8704) (83.589, -173.2305) (83.4587, -173.5115) (83.367, -173.7129) (83.3124, -173.834) (83.2942, -173.8747) knots -1 -1 -1 -1 -1 -1 -0.98571429 -0.97142857 -0.95714286 -0.94285714 -0.92857143 -0.91428571 -0.9 -0.88571429 -0.87142857 -0.85714286 -0.84285714 -0.82857143 -0.81428571 -0.8 -0.78571429 -0.77142857 -0.75714286 -0.74285714 -0.72857143 -0.71428571 -0.7 -0.68571429 -0.67142857 -0.65714286 -0.64285714 -0.62857143 -0.61428571 -0.6 -0.58571429 -0.57142857 -0.55714286 -0.54285714 -0.52857143 -0.51428571 -0.5 -0.48571429 -0.47142857 -0.45714286 -0.44285714 -0.42857143 -0.41428571 -0.4 -0.38571429 -0.37142857 -0.35714286 -0.34285714 -0.32857143 -0.31428571 -0.3 -0.28571429 -0.27142857 -0.25714286 -0.24285714 -0.22857143 -0.21428571 -0.2 -0.18571429 -0.17142857 -0.15714286 -0.14285714 -0.12857143 -0.11428571 -0.10707295 -0.10707295 -0.10707295 -0.10707295 -0.10707295 -0.10707295
  spline S131 degree 3 poles (81.438, -174.7588) (81.6377, -174.812) (81.846, -174.8255) (82.256, -174.7721) (82.4538, -174.7056) (82.7783, -174.5203) (82.9093, -174.415) (83.1338, -174.1677) (83.2258, -174.027) (83.2942, -173.8747) knots 0 0 0 0 0.062015 0.062015 0.12403 0.12403 0.174133 0.174133 0.224236 0.224236 0.224236 0.224236
  arc A66 (81.438, -174.7588) -> (73.3043, -172.7309) centre (11.949, -436.1388) ccw
  spline S132 degree 3 poles (72.0805, -171.0788) (72.0667, -171.2851) (72.0933, -171.492) (72.2244, -171.8841) (72.3276, -172.0655) (72.5718, -172.3484) (72.7002, -172.4569) (72.986, -172.6297) (73.1417, -172.693) (73.3043, -172.7309) knots 0 0 0 0 0.062015 0.062015 0.12403 0.12403 0.174133 0.174133 0.224236 0.224236 0.224236 0.224236
  spline S133 degree 5 poles (72.0805, -171.0788) (72.0835, -171.0343) (72.0922, -170.9017) (72.1057, -170.6809) (72.1226, -170.3716) (72.141, -169.9735) (72.1577, -169.5312) (72.1709, -169.0885) (72.1807, -168.6454) (72.187, -168.2019) (72.19, -167.7579) (72.1895, -167.3136) (72.1856, -166.8688) (72.1786, -166.4237) (72.1684, -165.9783) (72.1553, -165.5326) (72.1394, -165.0866) (72.1207, -164.6404) (72.0992, -164.1939) (72.075, -163.7473) (72.0482, -163.3003) (72.0188, -162.8532) (71.9867, -162.4059) (71.9521, -161.9584) (71.915, -161.5108) (71.8754, -161.063) (71.8335, -160.615) (71.7891, -160.1669) (71.7425, -159.7187) (71.6935, -159.2704) (71.6422, -158.8219) (71.5887, -158.3734) (71.533, -157.9247) (71.475, -157.476) (71.4149, -157.0272) (71.3526, -156.5783) (71.2882, -156.1294) (71.2216, -155.6804) (71.153, -155.2313) (71.0824, -154.7823) (71.0097, -154.3331) (70.9349, -153.884) (70.8582, -153.4348) (70.7794, -152.9856) (70.6987, -152.5364) (70.6161, -152.0872) (70.5315, -151.638) (70.445, -151.1888) (70.3566, -150.7396) (70.2662, -150.2905) (70.1741, -149.8413) (70.08, -149.3922) (69.9841, -148.9431) (69.8864, -148.494) (69.7869, -148.045) (69.6855, -147.596) (69.5824, -147.1471) (69.4774, -146.6983) (69.3707, -146.2495) (69.2623, -145.8007) (69.1521, -145.352) (69.0401, -144.9035) (68.9265, -144.4549) (68.8111, -144.0065) (68.7174, -143.6478) (68.6464, -143.3788) (68.5987, -143.1995) (68.5748, -143.1099) knots 0.10707295 0.10707295 0.10707295 0.10707295 0.10707295 0.10707295 0.11428571 0.12857143 0.14285714 0.15714286 0.17142857 0.18571429 0.2 0.21428571 0.22857143 0.24285714 0.25714286 0.27142857 0.28571429 0.3 0.31428571 0.32857143 0.34285714 0.35714286 0.37142857 0.38571429 0.4 0.41428571 0.42857143 0.44285714 0.45714286 0.47142857 0.48571429 0.5 0.51428571 0.52857143 0.54285714 0.55714286 0.57142857 0.58571429 0.6 0.61428571 0.62857143 0.64285714 0.65714286 0.67142857 0.68571429 0.7 0.71428571 0.72857143 0.74285714 0.75714286 0.77142857 0.78571429 0.8 0.81428571 0.82857143 0.84285714 0.85714286 0.87142857 0.88571429 0.9 0.91428571 0.92857143 0.94285714 0.95714286 0.97142857 0.98571429 1 1 1 1 1 1
  arc A67 (68.5748, -143.1099) -> (58.96, -141.4145) centre (11.949, -436.1388) ccw